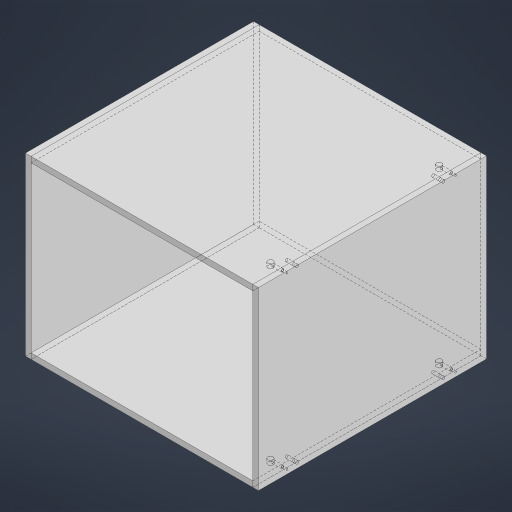
# Autodesk Inventor part: Деталь1
Saved by Autodesk Inventor 2023.4 (Build 274418000, 418)
## iProperties
Created: 2026-09-26
Part Number: Деталь1
Material: Типовые
Document SubType Name: Modeling
Designer: desig
Density: 1 g/cm^3
Appearance: По умолчанию
Author: desig
Autodesk Inventor part; units mm, degrees
ref_plane "YZ Plane" through (0, 0, 0) normal (1, 0, 0) x (0, 1, 0)
ref_plane "XZ Plane" through (0, 0, 0) normal (0, 1, 0) x (-1, 0, 0)
ref_plane "XY Plane" through (0, 0, 0) normal (0, 0, 1) x (1, 0, 0)
sketch "Эскиз1" plane through (0, 0, 0) normal (0, 1, 0) x (-1, 0, 0)
  line L0 (0, 0) -> (-16, 0)
  line L1 (-16, 0) -> (-16, -648.6531)
  line L2 (-16, -648.6531) -> (0, -648.6531)
  line L3 (0, -648.6531) -> (0, 0)
  line L4 (-646.4743, 0) -> (-662.4743, 0)
  line L5 (-662.4743, 0) -> (-662.4743, -648.6531)
  line L6 (-662.4743, -648.6531) -> (-646.4743, -648.6531)
  line L7 (-646.4743, -648.6531) -> (-646.4743, 0)
  line L8 (-16, -648.6531) -> (-646.4743, -648.6531)
  line L9 (-16, 0) -> (-646.4743, 0)
  dimension "d0" = 16
  dimension "d1" = 16
  dimension "d46" = 648.653
  dimension "d47" = 662.474
  constraints: 20 end point, 4 parallel, 3 horizontal, 3 perpendicular, 2 point on line
  measures "d0" distance of L1.end L2.end
  measures "d1" distance of L5.end L6.end
  measures "d46" distance of L2.end L0.start
  measures "d47" distance between parallel lines of L5 L3
extrude "Выдавливание1" add sketch "Эскиз1" along normal blind 500 contours L3 L2 L1 L0
extrude "Выдавливание2" add sketch "Эскиз1" against normal blind 16 from surface at 500 separate body contours L1 L8 L7 L9
extrude "Выдавливание3" add sketch "Эскиз1" along normal blind 16 separate body contours L1 L8 L7 L9
extrude "Выдавливание4" add sketch "Эскиз1" along normal up to surface (500 mm away) separate body contours L7 L6 L5 L4
sketch "DrillingSketch_1" plane through (646.4743, 484, -648.6531) normal (1, 0, 0) x (0, 0, -1)
  line L0 (0, 0) -> (-648.6531, 0) projected
  line L1 (0, 0) -> (0, 16) projected
  line L2 (0, 16) -> (-648.6531, 16) projected
  line L3 (-648.6531, 0) -> (-648.6531, 16) projected
  line L4 (0, 8) -> (-648.6531, 8) construction
  line L5 (-324.3266, 8) -> (-324.3266, -12) construction
  line L6 (-648.6531, -484) -> (0, -484) projected
  line L7 (0, -484) -> (0, -468) projected
  line L8 (-648.6531, -468) -> (0, -468) projected
  line L9 (-648.6531, -484) -> (-648.6531, -468) projected
  line L10 (0, -476) -> (-648.6531, -476) construction
  line L11 (-324.3266, -476) -> (-324.3266, -496) construction
  point P0 (-84.3266, 8)
  point P1 (-564.3266, 8)
  point P2 (-116.3266, 8)
  point P3 (-532.3266, 8)
  point P4 (-84.3266, -476)
  point P5 (-564.3266, -476)
  point P6 (-116.3266, -476)
  point P7 (-532.3266, -476)
  dimension "d5" = 16
  dimension "d6" = 0
  dimension "Минимальный_отступ_присадки_от_кромки_Каркас" = 70
  dimension "Long_edge_1" = 648.6531
  dimension "Расстояние_между_точками" = 480
  dimension "d2457" = 32
  dimension "Long_edge_2" = 648.6531
  dimension "Расстояние_между_точками_2" = 480
  dimension "d2460" = 32
  constraints: 10 point on line, 8 end point, 8 midpoint, 4 symmetric about line, 2 perpendicular
  measures "Long_edge_1" distance of L4.start L4.end
  measures "Расстояние_между_точками" distance of point (-564.327, 8) point (-84.327, 8)
  measures "d2457" distance of point (-84.327, 8) point (-116.327, 8)
  measures "Long_edge_2" distance of L10.start L10.end
  measures "Расстояние_между_точками_2" distance of point (-564.327, -476) point (-84.327, -476)
  measures "d2460" distance of point (-84.327, -476) point (-116.327, -476)
hole "Stiajka outer 8x34" at (646.4743, 492, -564.3266) at (646.4743, 492, -84.3266) direction (-1, 0, 0) diameter 8 depth 34 bodies 1 2 3 4
hole "Stiajka outer 5x13" at (646.4743, 492, -564.3266) at (646.4743, 492, -84.3266) direction (1, 0, 0) diameter 5 depth 12.5 bodies 1 2 3 4
hole "Shkant 8x10" at (646.4743, 492, -532.3266) at (646.4743, 492, -116.3266) direction (1, 0, 0) diameter 8 depth 10 bodies 1 2 3 4
hole "Shkant 8x20" at (646.4743, 492, -532.3266) at (646.4743, 492, -116.3266) direction (-1, 0, 0) diameter 8 depth 20 bodies 1 2 3 4
sketch "StiajkaSideSketch" plane through (16, 484, 0) normal (0, -1, 0) x (1, 0, 0)
  line L0 (630.4743, -560.3266) -> (630.4743, -568.3266) projected
  line L1 (596.4743, -568.3266) -> (596.4743, -560.3266) projected
  line L2 (630.4743, -80.3266) -> (630.4743, -88.3266) projected
  line L3 (596.4743, -88.3266) -> (596.4743, -80.3266) projected
  point P0 (596.4743, -564.3266)
  point P1 (596.4743, -84.3266)
  dimension "d46" = 648.653
  dimension "d47" = 662.474
  dimension "Минимальный_отступ_присадки_от_кромки_Каркас" = 70
  constraints: 2 midpoint
hole "Stiajka cup" at (612.4743, 484, -564.3266) at (612.4743, 484, -84.3266) direction (0, 1, 0) diameter 15 depth 12.5 bodies 1 2 3 4
hole "Stiajka outer 8x34 2" at (646.4743, 8, -564.3266) at (646.4743, 8, -84.3266) direction (-1, 0, 0) diameter 8 depth 34 bodies 1 2 3 4
hole "Stiajka outer 5x13 2" at (646.4743, 8, -564.3266) at (646.4743, 8, -84.3266) direction (1, 0, 0) diameter 5 depth 12.5 bodies 1 2 3 4
hole "Shkant 8x10 2" at (646.4743, 8, -532.3266) at (646.4743, 8, -116.3266) direction (1, 0, 0) diameter 8 depth 10 bodies 1 2 3 4
hole "Shkant 8x20 2" at (646.4743, 8, -532.3266) at (646.4743, 8, -116.3266) direction (-1, 0, 0) diameter 8 depth 20 bodies 1 2 3 4
sketch "StiajkaSideSketch_2" plane through (0, 0, 0) normal (0, -1, 0) x (1, 0, 0)
  line L0 (646.4743, -560.3266) -> (646.4743, -568.3266) projected
  line L1 (612.4743, -568.3266) -> (612.4743, -560.3266) projected
  line L2 (646.4743, -80.3266) -> (646.4743, -88.3266) projected
  line L3 (612.4743, -88.3266) -> (612.4743, -80.3266) projected
  point P0 (612.4743, -564.3266)
  point P1 (612.4743, -84.3266)
  dimension "d46" = 648.653
  dimension "d47" = 662.474
  dimension "Минимальный_отступ_присадки_от_кромки_Каркас" = 70
  constraints: 2 midpoint
hole "Stiajka cup 2" at (612.4743, 0, -564.3266) at (612.4743, 0, -84.3266) direction (0, 1, 0) diameter 15 depth 12.5 bodies 1 2 3 4
equation "\"d0\" = Толщина_каркаса"
equation "\"d1\" = Толщина_каркаса"
equation "\"d5\" = Толщина_каркаса"
equation "\"d7\" = Толщина_каркаса"
equation "\"Минимальный_отступ_присадки_от_кромки_Каркас\" = 70"
equation "\"Толщина_каркаса\" = 16"
equation "\"Стяжка_D\" = 15"
equation "\"Стяжка_h\" = 12.5"
equation "\"Стяжка_D_резьбыШтока\" = 5"
equation "\"Стяжка_D_телаШтока\" = 8"
equation "\"Стяжка_резьбыШтока_Петля_h\" = 12.5"
equation "\"Стяжка_отступ\" = 34"
equation "\"Конфирмат_D_вПласть\" = 8"
equation "\"Конфирмат_D_вТорец\" = 5"
equation "\"Толщина_каркаса_ящика\" = 16"
equation "\"Шкант_D\" = 8"
equation "\"Полкодержатель_D\" = 5"
equation "\"Полкодержатель_смещение_от_низа_полки\" = 5"
equation "\"Петля_D_присадки\" = 35"
equation "\"M_Конфирмат_глубина_резьбы\" = 35"
equation "\"M_Конфирмат_D_вПласть\" = 5"
equation "\"M_Конфирмат_D_вТорец\" = 3"
equation "\"Толщина_задн_ст_Володя\" = 3"
equation "\"Толщина_дна_ящика_Володя\" = 6"
equation "\"Минимальное_расстояния_от_заднСт_ящика_до_заднСт\" = 25"
equation "\"Западание_кромки_полки_за_каркас\" = 5"
